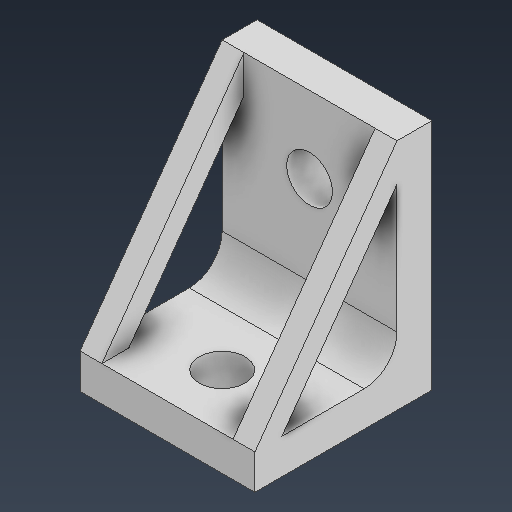
# Autodesk Inventor part: мертвое колесо крепл 25-26
Saved by Autodesk Inventor 2026 (Build 300175000, 175)
## iProperties
Created: 2025-09-25
Part Number: мертвое колесо крепл 25-26
Material: Типовые
Document SubType Name: Modeling
Designer: GameHD
Density: 1 g/cm^3
Appearance: По умолчанию
Author: GameHD
Autodesk Inventor part; units mm, degrees
ref_plane "YZ Plane" through (0, 0, 0) normal (1, 0, 0) x (0, 1, 0)
ref_plane "XZ Plane" through (0, 0, 0) normal (0, 1, 0) x (-1, 0, 0)
ref_plane "XY Plane" through (0, 0, 0) normal (0, 0, 1) x (1, 0, 0)
sketch "Эскиз1" plane through (0, 0, 0) normal (0, 0, 1) x (1, 0, 0)
  circle A0 centre (0, 0) radius 2.1
  line L0 (-5, 14.35) -> (5, 14.35)
  line L1 (5, 14.35) -> (5, -14.35)
  line L2 (5, -14.35) -> (-5, -14.35)
  line L3 (-5, -14.35) -> (-5, 14.35)
  line L4 (-5, 14.35) -> (5, -14.35) construction
  line L5 (5, 14.35) -> (-5, -14.35) construction
  line L6 (-5, 7) -> (5, 7)
  dimension "d0" = 4.2
  dimension "d2" = 10
  dimension "d3" = 28.7
  dimension "d4" = 7
  constraints: 14 end point, 2 midpoint, 2 parallel, 2 perpendicular, 2 point on line, 1 centre point, 1 coincident, 1 horizontal
  measures "d0" diameter of A0
  measures "d2" distance of L1.end L2.end
  measures "d3" distance of L2.end L0.start
  measures "d4" distance from line of A0.centre L6
extrude "Выдавливание1" add sketch "Эскиз1" along normal blind 3.2 contours L6 L1 L2 L3
sketch "Эскиз2" plane through (0, 0, 3.2) normal (0, 0, 1) x (1, 0, 0)
  line L0 (5, -14.35) -> (5, 7) projected
  line L1 (5, -14.35) -> (-5, -14.35)
  line L2 (-5, -14.35) -> (-5, -11.15)
  line L3 (-5, -11.15) -> (5, -11.15)
  line L4 (5, -11.15) -> (5, -14.35)
  point P0 (0, 0)
  point P1 (5, -11.15)
  dimension "d7" = 10
  dimension "d8" = 3.2
  constraints: 8 end point, 2 parallel, 1 horizontal, 1 perpendicular
  measures "d7" distance of L2.end L3.end
  measures "d8" distance of L1.end L2.end
extrude "Выдавливание2" add sketch "Эскиз2" along normal blind 13
fillet "Сопряжение1" radius 3 1 edges at (0, -11.15, 3.2)
sketch "Эскиз3" plane through (-5, -11.15, 16.2) normal (0, 1, 0) x (1, 0, 0)
  line L0 (0, 10) -> (10, 10) projected
  line L1 (5, 10) -> (5, 0)
  line L2 (0, 0) -> (10, 0) projected
  circle A0 centre (5, 5) radius 2.1
  point P0 (5, 16.2)
  dimension "d12" = 4.2
  constraints: 3 midpoint, 2 end point, 1 centre point
  measures "d12" diameter of A0
extrude "Выдавливание3" cut sketch "Эскиз3" against normal blind 13
sketch "Эскиз4" plane through (5, -14.35, 0) normal (1, 0, 0) x (0, 0, -1)
  line L0 (0, 0) -> (0, 21.35) projected
  line L1 (0, 21.35) -> (-3.2, 21.35) projected
  line L2 (-3.2, 6.2) -> (-3.2, 21.35) projected
  arc A0 (-6.2, 3.2) -> (-3.2, 6.2) centre (-6.2, 6.2) ccw projected
  line L3 (-6.2, 3.2) -> (-16.2, 3.2) projected
  line L4 (-16.2, 0) -> (-16.2, 3.2) projected
  line L5 (0, 0) -> (-16.2, 0) projected
  point P0 (0, 14.35)
extrude "Выдавливание4" add sketch "Эскиз4" along normal blind 3
sketch "Эскиз5" plane through (-5, -14.35, 0) normal (-1, 0, 0) x (0, 0, 1)
  line L0 (0, 21.35) -> (0, 0) projected
  line L1 (0, 0) -> (16.2, 0) projected
  line L2 (16.2, 3.2) -> (16.2, 0) projected
  line L3 (6.2, 3.2) -> (16.2, 3.2) projected
  arc A0 (3.2, 6.2) -> (6.2, 3.2) centre (6.2, 6.2) ccw projected
  line L4 (3.2, 21.35) -> (3.2, 6.2) projected
  line L5 (0, 21.35) -> (3.2, 21.35) projected
  point P0 (0, 14.35)
extrude "Выдавливание5" add sketch "Эскиз5" along normal blind 3
sketch "Эскиз6" plane through (8, -14.35, 0) normal (1, 0, 0) x (0, 0, -1)
  line L0 (-16.2, 3.2) -> (-16.2, 0) projected
  line L1 (-3.2, 21.35) -> (-16.2, 3.2)
  line L2 (-1.574, 20.1854) -> (-14.2, 2.5576)
  line L3 (-14.2, 2.5576) -> (-14.2, 0)
  line L4 (0, 0) -> (-16.2, 0) projected
  line L5 (0, 0) -> (0, 21.35) projected
  line L6 (0, 21.35) -> (-3.2, 21.35) projected
  line L7 (-3.2, 21.35) -> (-3.2, 6.2) projected
  arc A0 (-6.2, 3.2) -> (-3.2, 6.2) centre (-6.2, 6.2) ccw projected
  line L8 (-6.2, 3.2) -> (-16.2, 3.2) projected
  line L9 (-16.2, 3.2) -> (-16.2, 0) projected
  line L10 (-16.2, 0) -> (0, 0) projected
  point P0 (0, 14.35)
  point P1 (-13.7399, 3.2)
  point P2 (-3.2, 17.9153)
  dimension "d19" = 2
  constraints: 6 end point, 1 other
  measures "d19" distance between parallel lines of L1 L2
extrude "Выдавливание6" add sketch "Эскиз6" against normal blind 2 contours L1 L7 L2 L8
sketch "Эскиз7" plane through (-8, -14.35, 0) normal (-1, 0, 0) x (0, 0, 1)
  line L0 (16.2, 3.2) -> (13.7399, 3.2) projected
  line L1 (16.2, 3.2) -> (3.2, 21.35) projected
  line L2 (3.2, 17.9153) -> (3.2, 21.35) projected
  line L3 (3.2, 17.9153) -> (13.7399, 3.2) projected
  point P0 (0, 14.35)
extrude "Выдавливание7" add sketch "Эскиз7" against normal blind 2
